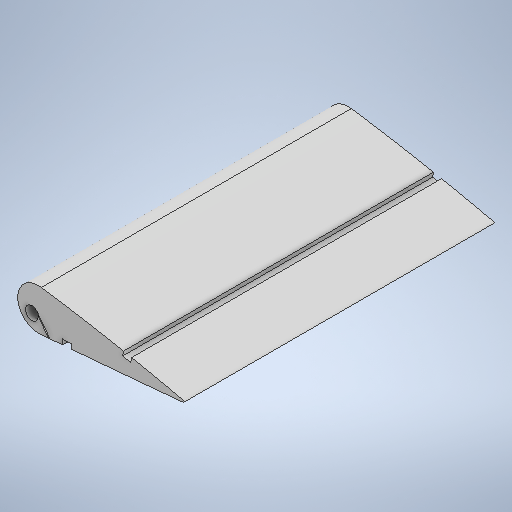
# Autodesk Inventor part: 2P.03.01.01.IM.FlapBody
Saved by Autodesk Inventor 2025.2 (Build 292293000, 293)
## iProperties
Created: 2024-12-30
Part Number: 2P.03.01.01.IM.FlapBody
Material: Generic
Document SubType Name: Modeling
Designer: Imist
Density: 1 g/cm^3
Appearance: Default
Author: Imist
Autodesk Inventor part; units mm, degrees
ref_plane "YZ Plane" through (0, 0, 0) normal (1, 0, 0) x (0, 1, 0)
ref_plane "XZ Plane" through (0, 0, 0) normal (0, 1, 0) x (-1, 0, 0)
ref_plane "XY Plane" through (0, 0, 0) normal (0, 0, 1) x (1, 0, 0)
sketch "Sketch2" plane through (0, 0, 0) normal (0, 0, 1) x (1, 0, 0)
  line L0 (18.7124, 8.328) -> (18.1325, 5.3846)
  line L1 (13.7124, 9.3131) -> (18.7124, 8.328)
  line L2 (13.1325, 6.3697) -> (13.7124, 9.3131)
  line L3 (18.1325, 5.3846) -> (13.1325, 6.3697)
  spline S0 degree 4 poles (-37.1669, 18.0129) (-32.0265, 17.2427) (-23.4508, 15.9354) (-12.1298, 14.0656) (1.57, 11.6269) (12.5569, 9.5628) (22.3152, 7.6138) (30.7628, 5.8944) (37.7432, 4.3297) (44.5535, 2.9574) (48.5705, 1.7508) (51.0887, 1.6849) (51.3931, 0.8429) knots 0 0 0 0 0 0.183688 0.302378 0.416104 0.523956 0.624947 0.717922 0.80148 0.873691 1 1 1 1 1
  spline S1 degree 2 poles (-25.5966, 10.0026) (-25.4878, 9.9865) (-25.3792, 9.9704) knots 0 0 0 1 1 1
  line L4 (-25.4014, 9.9736) -> (-25.357, 9.9671) construction
  arc A0 (-25.3615, 9.9677) -> (-25.3969, 9.973) centre (-40.9588, -94.8535) ccw construction
  line L5 (-24.2835, -3.2624) -> (-24.0359, -6.2521)
  line L6 (-24.0359, -6.2521) -> (-18.3701, -5.783)
  line L7 (-18.6176, -2.7932) -> (-24.2835, -3.2624)
  line L8 (-39.0627, 5.3599) -> (-39.0627, 1.3599)
  line L9 (-39.0627, 1.3599) -> (-43.0627, 1.3599)
  arc A1 (-39.8677, 3.7666) -> (-39.0627, 1.3682) centre (-43.0627, 1.3599) ccw
  arc A2 (-37.1669, 18.0129) -> (-38.0249, -7.3921) centre (-39.0627, 5.3599) ccw
  line L10 (-18.3701, -5.783) -> (-18.6176, -2.7932)
  spline S2 degree 4 poles (9.4193, -3.4138) (11.4228, -3.2393) (15.865, -2.8497) (22.3591, -2.2688) (30.3236, -1.5742) (37.4254, -0.8702) (44.3418, -0.3579) (48.4757, 0.3135) (50.9779, 0.0538) (51.3931, 0.8429) knots 0.442408 0.442408 0.442408 0.442408 0.442408 0.523404 0.624432 0.717481 0.801136 0.873452 1 1 1 1 1
  line L11 (4.7469, -3.8205) -> (14.0918, -3.007) construction
  arc A3 (5.6813, -3.7375) -> (13.1571, -3.0867) centre (-353.4721, 4165.1771) ccw construction
  line L12 (-18.3701, -5.783) -> (-10.8502, -5.1603) construction
  line L13 (-10.8502, -5.1603) -> (1.3894, -4.1468) construction
  line L14 (1.3894, -4.1468) -> (12.5371, -3.1411) construction
  spline S3 degree 3 poles (-18.3701, -5.783) (-10.8502, -5.1603) (1.3894, -4.1468) (12.5371, -3.1411) knots 1 1 1 1 2 2 2 2
  line L15 (-39.8677, 3.7666) -> (-31.8412, -6.8892)
  line L16 (-39.0627, 1.3682) -> (-32.7849, -6.9659)
  spline S4 degree 4 poles (-38.0249, -7.3921) (-36.8101, -7.2933) (-35.4821, -7.1853) (-34.1239, -7.0749) (-32.7849, -6.9659) knots 0 0 0 0 0 1 1 1 1 1
  spline S5 degree 4 poles (-31.8412, -6.8892) (-27.1613, -6.5084) (-22.9298, -6.1633) (-21.0796, -6.0088) (-18.3701, -5.783) knots 0.24985 0.24985 0.24985 0.24985 0.24985 1 1 1 1 1
  line L17 (-33.3312, -7.0104) -> (-32.2386, -6.9215) construction
  arc A4 (-33.2219, -7.0015) -> (-32.3479, -6.9304) centre (-843.5448, 9960.1133) ccw construction
  line L18 (-33.4282, -7.0183) -> (-30.2541, -6.76) construction
  arc A5 (-33.1108, -6.9924) -> (-30.5716, -6.7858) centre (-842.8237, 9960.172) ccw construction
  point P0 (0, 0)
  point P1 (0.9282, 3.5218)
  point P2 (-2.5419, 1.8477)
  point P3 (-23.1779, 15.8549)
  point P4 (-10.0259, 13.6649)
  point P5 (2.1391, 11.4989)
  point P6 (13.1941, 9.4139)
  point P7 (23.0191, 7.4639)
  point P8 (31.5091, 5.7029)
  point P9 (38.5801, 4.1789)
  point P10 (44.1541, 2.9429)
  point P11 (48.1801, 2.0309)
  point P12 (50.6101, 1.4729)
  point P13 (-10.8502, -5.1603)
  point P14 (1.3894, -4.1468)
  point P15 (31.0831, -1.4851)
  point P16 (38.2711, -0.8281)
  point P17 (43.9471, -0.3001)
  point P18 (48.0511, 0.0869)
  point P19 (50.5321, 0.3239)
  point P20 (-51.8495, 5.7955)
  point P21 (51.3931, 1.2839)
  point P22 (-51.8489, 20.0789)
  point P23 (-52.6589, -8.5531)
  point P24 (51.3931, 0.4019)
  point P25 (-37.1669, 5.3448)
  point P26 (-23.1779, 4.8372)
  point P27 (-10.0259, 4.2921)
  point P28 (2.1391, 3.7285)
  point P29 (13.1941, 3.1654)
  point P30 (23.0191, 2.6255)
  point P31 (31.5091, 2.1283)
  point P32 (38.5801, 1.6897)
  point P33 (44.1541, 1.3311)
  point P34 (48.1801, 1.065)
  point P35 (50.6101, 0.9019)
  point P36 (-25.9398, -0.159)
  point P37 (9.8274, 3.135)
  point P38 (-20.001, 9.1398)
  point P39 (-14.7402, 8.2638)
  point P40 (-9.8742, 7.3974)
  point P41 (-5.4522, 6.5634)
  point P42 (-1.5222, 5.7834)
  point P43 (1.8738, 5.079)
  point P44 (4.7022, 4.4694)
  point P45 (6.9318, 3.975)
  point P46 (8.5422, 3.6102)
  point P47 (9.5142, 3.387)
  point P48 (-20.3442, 0.297)
  point P49 (-15.0702, 0.7374)
  point P50 (-10.1754, 1.155)
  point P51 (-5.715, 1.5414)
  point P52 (-1.7406, 1.893)
  point P53 (1.7034, 2.2038)
  point P54 (4.5786, 2.4666)
  point P55 (6.849, 2.6778)
  point P56 (8.4906, 2.8326)
  point P57 (9.483, 2.9274)
  point P58 (9.4193, -3.4138)
  point P59 (-39.0627, 1.3682)
  point P60 (-39.0627, 1.3599)
  dimension "d14" = 3
  dimension "d15" = 5
  dimension "d16" = 52.7751
  dimension "d17" = 3
  dimension "d18" = 5.6658
  dimension "d19" = 4
  dimension "d20" = 4
  dimension "d21" = 8
  dimension "d23" = 0.8
  constraints: 32 end point, 9 point on circle, 8 midpoint, 6 centre point, 5 parallel, 3 coincident, 3 perpendicular, 1 point on line, 1 tangent, 1 vertical, 43 other
  measures "d14" distance of L0.start L0.end
  measures "d15" horizontal distance of L0.start L1.start
  measures "d16" horizontal distance of L8.start L1.start
  measures "d17" distance of L7.start L10.start
  measures "d18" horizontal distance of L7.start L5.start
  measures "d19" distance of L8.start L8.end
  measures "d20" distance of L8.end L9.end
  measures "d21" diameter of A1
  measures "d23" distance between parallel lines of L15 L16
extrude "Extrusion3" add sketch "Sketch2" along normal blind 192 contours S0 S2 S3 L10 L7 L5 S5 L15 A1 L8 L16 S4 A2 L2 L3 L0
body "Solid3"
